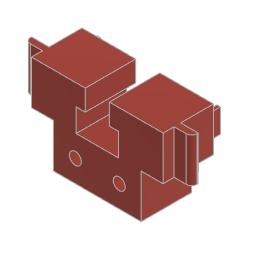
belt tensioner spacer (Autodesk Fusion 360 design; units mm, degrees)
Autodesk Fusion 360 part; units mm, degrees
sketch "Sketch1" plane through (0, 0, 0) normal (0, 1, 0) x (1, 0, 0)
  line L0 (0, 0) -> (0, -20) construction
  line L1 (0, -20) -> (30, -20)
  line L2 (30, -20) -> (30, 0)
  line L3 (30, 0) -> (20, 0)
  line L4 (20, 0) -> (20, 20)
  line L5 (20, 20) -> (0, 20)
  line L6 (-20, 0) -> (-20, 20)
  line L7 (-30, 0) -> (-20, 0)
  line L8 (-30, -20) -> (-30, 0)
  line L9 (-20, 20) -> (0, 20)
  line L10 (0, -20) -> (-30, -20)
  dimension "d1" = 20
  dimension "d2" = 30
  constraint coincident L0.start origin
  constraint vertical L0
  constraint perpendicular L0 L1
  constraint perpendicular L1 L2
  constraint perpendicular L2 L3
  constraint perpendicular L3 L4
  constraint perpendicular L4 L5
  constraint symmetric L1.start L0 L10.start
  constraint symmetric L0 L1.end L8.start
  constraint symmetric L0 L2.end L7.start
  constraint symmetric L0 L3.end L6.start
  constraint symmetric L0 L4.end L6.end
  constraint symmetric L0 L5.end L9.end
  measures "d1" distance of L0.start L0.end
  measures "d2" distance of L0.end L1.end
extrude "Extrude1" add sketch "Sketch1" along normal blind 15
sketch "Sketch2" plane through (0, 0, 0) normal (0, -1, 0) x (1, 0, 0)
  line L0 (30, 0) -> (30, 20)
  line L1 (30, 20) -> (-30, 20)
  line L2 (-30, 20) -> (-30, 0)
  line L3 (-30, 0) -> (-20, 0)
  line L4 (-20, 0) -> (-20, -20)
  line L5 (-20, -20) -> (20, -20)
  line L6 (20, -20) -> (20, 0)
  line L7 (20, 0) -> (30, 0)
  line L8 (30, 20) -> (38, 20)
  line L9 (38, 20) -> (38, 0)
  line L10 (38, 0) -> (30, 0)
  line L11 (30, 0) -> (30, 20)
  line L12 (-30, 20) -> (-38, 20)
  line L13 (-38, 20) -> (-38, 0)
  line L14 (-38, 0) -> (-30, 0)
  line L15 (-30, 0) -> (-30, 20)
  dimension "d5" = 8
  dimension "d6" = 8
  dimension "d7" = 20
  constraint horizontal L8
  constraint vertical L9
  constraint horizontal L10
  constraint vertical L11
  constraint coincident L0.end L1.start
  constraint horizontal L12
  constraint vertical L13
  constraint horizontal L14
  constraint vertical L15
  constraint coincident L1.end L2.start
  measures "d5" distance of L0.end L8.end
  measures "d6" distance of L1.end L12.end
  measures "d7" distance of L1.end L2.end
extrude "Extrude2" add sketch "Sketch2" along normal blind 3
sketch "Sketch3" plane through (0, -3, 0) normal (0, -1, 0) x (1, 0, 0)
  line L0 (38, 20) -> (-38, 20)
  line L1 (-38, 20) -> (-38, 0)
  line L2 (-38, 0) -> (-20, 0)
  line L3 (-20, 0) -> (-20, -20)
  line L4 (-20, -20) -> (20, -20)
  line L5 (20, -20) -> (20, 0)
  line L6 (20, 0) -> (38, 0)
  line L7 (38, 0) -> (38, 20)
  line L8 (-30, 20) -> (-30, 0)
  line L9 (0, 20) -> (-30, 20)
  line L10 (30, 20) -> (30, 0)
  line L11 (0, 20) -> (30, 20)
  line L12 (30, 0) -> (20, 0)
  line L13 (20, 0) -> (20, -20)
  line L14 (20, -20) -> (0, -20)
  line L15 (-20, -20) -> (0, -20)
  line L16 (-20, 0) -> (-20, -20)
  line L17 (-30, 0) -> (-20, 0)
extrude "Extrude3" add sketch "Sketch3" along normal blind 5 contours L0 L2 L3 L4 L5 L6 L8 L9 L10 L11 L12 L13 L14 L15 L16 L17
fillet "Fillet1" radius 2.5 2 edges at (38, -3, 10) (-38, -3, 10)
sketch "Sketch4" plane through (0, -8, 0) normal (0, -1, 0) x (1, 0, 0)
  line L0 (30, 20) -> (-30, 20)
  line L1 (-30, 20) -> (-30, 0)
  line L2 (-30, 0) -> (-20, 0)
  line L3 (-20, 0) -> (-20, -20)
  line L4 (-20, -20) -> (20, -20)
  line L5 (20, -20) -> (20, 0)
  line L6 (20, 0) -> (30, 0)
  line L7 (30, 0) -> (30, 20)
  line L8 (-20, -10) -> (20, -10) construction
  line L9 (20, 0) -> (20, -20)
  line L10 (-5.5, 20) -> (0, 20)
  line L11 (0, 20) -> (0, 13.9)
  line L12 (0, 13.9) -> (-5.5, 13.9)
  line L13 (-5.5, 13.9) -> (-5.5, 20)
  line L14 (0, 13.9) -> (5.5, 13.9)
  line L15 (5.5, 13.9) -> (5.5, 20)
  line L16 (5.5, 20) -> (0, 20)
  line L17 (14.8575, 20) -> (-15.1425, 20)
  line L18 (-15.1425, 20) -> (-15.1425, 10.5)
  line L19 (-15.1425, 10.5) -> (14.8575, 10.5)
  line L20 (14.8575, 10.5) -> (14.8575, 20)
  line L21 (14.8575, 20) -> (-15.1425, 10.5) construction
  line L22 (-15.1425, 20) -> (14.8575, 10.5) construction
  line L23 (9.65, 0) -> (-9.65, 0)
  line L24 (-9.65, 0) -> (-9.65, 10.5)
  line L25 (-9.65, 10.5) -> (9.65, 10.5)
  line L26 (9.65, 10.5) -> (9.65, 0)
  line L27 (9.65, 0) -> (-9.65, 10.5) construction
  line L28 (-9.65, 0) -> (9.65, 10.5) construction
  line L29 (5.5, 13.9) -> (14.8575, 13.9)
  line L30 (-15.1425, 13.9) -> (-5.5, 13.9)
  line L31 (-5.5, 13.9) -> (-5.5, 10.5)
  line L32 (5.5, 13.9) -> (5.5, 10.5)
  point P0 (-10, -10)
  point P1 (10, -10)
  point P2 (-0.1425, 15.25)
  point P3 (0, 5.25)
  dimension "d14" = 10
  dimension "d15" = 10
  dimension "d19" = 5.5
  dimension "d20" = 6.1
  dimension "d21" = 24.5
  dimension "d37" = 30
  dimension "d38" = 9.5
  dimension "d39" = 19.3
  dimension "d40" = 10.5
  constraint midpoint L3 L8.start
  constraint midpoint L5 L8.end
  constraint coincident L8 P0
  constraint coincident L8 P1
  constraint horizontal L10
  constraint vertical L11
  constraint horizontal L12
  constraint vertical L13
  constraint coincident L0 L10.start
  constraint symmetric L10.start L11 L15.end
  constraint symmetric L10.end L11 L16.end
  constraint symmetric L12.start L11 L14.start
  constraint symmetric L12.end L11 L14.end
  constraint horizontal L17
  constraint perpendicular L17 L18
  constraint parallel L17 L19
  constraint parallel L18 L20
  constraint coincident L21 P2
  constraint coincident L22 P2
  constraint collinear L0 L17
  constraint horizontal L23
  constraint perpendicular L23 L24
  constraint parallel L23 L25
  constraint parallel L24 L26
  constraint coincident L27 P3
  constraint coincident L28 P3
  constraint collinear L19 L25
  constraint coincident L20 L29.end
  constraint perpendicular L20 L29
  constraint coincident L18 L30.start
  constraint perpendicular L13 L30
  constraint coincident L25 L31.end
  constraint coincident L19 L32.end
  constraint vertical L32
  constraint vertical L31
  measures "d14" distance of L8.start P0
  measures "d15" distance of P1 L9
  measures "d19" distance of L11.end L12.end
  measures "d20" distance of L10.start L12.end
  measures "d21" distance of L0.end L13
  measures "d37" distance of L18.end L19.end
  measures "d38" distance of L17.end L18.end
  measures "d39" distance of L24.end L25.end
  measures "d40" distance of L23.end L24.end
hole "Hole1" at (10, -8, -10) at (-10, -8, -10) direction (0, 1, 0) diameter 5.5 end through all
extrude "Extrude4" cut sketch "Sketch4" against normal through all contours L0 L11 L14 L15 L16 L17 | L0 L10 L11 L12 L13 L17 | L12 L14 L19 L25 L31 L32 | L19 L23 L24 L25 L26
sketch "Sketch5" plane through (0, 15, 0) normal (0, 1, 0) x (-1, 0, 0)
  line L0 (-5.5, 20) -> (-30, 20)
  line L1 (-30, 20) -> (-30, 0)
  line L2 (-30, 0) -> (-20, 0)
  line L3 (-20, 0) -> (-20, -20)
  line L4 (-20, -20) -> (20, -20)
  line L5 (20, -20) -> (20, 0)
  line L6 (20, 0) -> (30, 0)
  line L7 (30, 0) -> (30, 20)
  line L8 (30, 20) -> (5.5, 20)
  circle A0 centre (-10, -10) radius 2.75
  circle A1 centre (10, -10) radius 2.75
  line L9 (0, 13.9) -> (0, -20) construction
  line L10 (-20, -10) -> (20, -10) construction
  line L11 (-16.55, -15.425) -> (-18.15, -15.425)
  line L12 (-18.15, -15.425) -> (-18.15, -4.575)
  line L13 (-18.15, -4.575) -> (-16.55, -4.575)
  line L14 (-16.55, -4.575) -> (-16.55, -15.425)
  line L15 (-16.55, -15.425) -> (-18.15, -4.575) construction
  line L16 (-18.15, -15.425) -> (-16.55, -4.575) construction
  line L17 (-13.95, -12.825) -> (-16.55, -12.825)
  line L18 (-16.55, -12.825) -> (-16.55, -7.175)
  line L19 (-16.55, -7.175) -> (-13.95, -7.175)
  line L20 (-13.95, -7.175) -> (-13.95, -12.825)
  line L21 (-13.95, -12.825) -> (-16.55, -7.175) construction
  line L22 (-16.55, -12.825) -> (-13.95, -7.175) construction
  line L23 (-16.55, -4.575) -> (-13.95, -7.175)
  line L24 (-13.95, -12.825) -> (-16.55, -15.425)
  line L25 (18.15, -4.575) -> (16.55, -4.575)
  line L26 (16.55, -4.575) -> (13.95, -7.175)
  line L27 (13.95, -7.175) -> (13.95, -12.825)
  line L28 (13.95, -12.825) -> (16.55, -15.425)
  line L29 (16.55, -15.425) -> (18.15, -15.425)
  line L30 (18.15, -15.425) -> (18.15, -4.575)
  line L31 (-30, 10) -> (30, 10) construction
  line L32 (-26.55, 4.575) -> (-28.15, 4.575)
  line L33 (-28.15, 4.575) -> (-28.15, 15.425)
  line L34 (-28.15, 15.425) -> (-26.55, 15.425)
  line L35 (-26.55, 15.425) -> (-26.55, 4.575)
  line L36 (-26.55, 4.575) -> (-28.15, 15.425) construction
  line L37 (-28.15, 4.575) -> (-26.55, 15.425) construction
  line L38 (-23.95, 7.175) -> (-26.55, 7.175)
  line L39 (-26.55, 7.175) -> (-26.55, 12.825)
  line L40 (-26.55, 12.825) -> (-23.95, 12.825)
  line L41 (-23.95, 12.825) -> (-23.95, 7.175)
  line L42 (-23.95, 7.175) -> (-26.55, 12.825) construction
  line L43 (-26.55, 7.175) -> (-23.95, 12.825) construction
  line L44 (-23.95, 12.825) -> (-26.55, 15.425)
  line L45 (-23.95, 7.175) -> (-26.55, 4.575)
  line L46 (23.95, 7.175) -> (26.55, 4.575)
  line L47 (23.95, 12.825) -> (23.95, 7.175)
  line L48 (23.95, 12.825) -> (26.55, 15.425)
  line L49 (28.15, 15.425) -> (26.55, 15.425)
  line L50 (28.15, 4.575) -> (28.15, 15.425)
  line L51 (26.55, 4.575) -> (28.15, 4.575)
  line L52 (5.5, 10.5) -> (9.65, 10.5)
  line L53 (9.65, 10.5) -> (9.65, 0)
  line L54 (9.65, 0) -> (-9.65, 0)
  line L55 (-9.65, 0) -> (-9.65, 10.5)
  line L56 (-9.65, 10.5) -> (-5.5, 10.5)
  line L57 (-5.5, 10.5) -> (-5.5, 20)
  line L58 (5.5, 20) -> (5.5, 10.5)
  point P0 (-17.35, -10)
  point P1 (-15.25, -10)
  point P2 (-27.35, 10)
  point P3 (-25.25, 10)
  dimension "d24" = 1.6
  dimension "d25" = 10.85
  dimension "d26" = 1.85
  dimension "d28" = 5.65
  dimension "d31" = 45
  dimension "d32" = 1.6
  dimension "d33" = 10.85
  dimension "d34" = 5.65
  dimension "d35" = 45
  dimension "d36" = 1.85
  constraint midpoint L4 L9.end
  constraint midpoint L3 L10.start
  constraint midpoint L5 L10.end
  constraint horizontal L11
  constraint perpendicular L11 L12
  constraint parallel L11 L13
  constraint parallel L12 L14
  constraint coincident L15 P0
  constraint coincident L16 P0
  constraint coincident L10 P0
  constraint horizontal L17
  constraint perpendicular L17 L18
  constraint parallel L17 L19
  constraint parallel L18 L20
  constraint coincident L21 P1
  constraint coincident L22 P1
  constraint coincident L10 P1
  constraint collinear L14 L18
  constraint symmetric L9 L11.start L28.end
  constraint symmetric L9 L11.end L29.end
  constraint symmetric L9 L12.end L25.start
  constraint symmetric L9 L13.end L25.end
  constraint symmetric L9 L17.start L27.end
  constraint symmetric L9 L19.end L26.end
  constraint midpoint L1 L31.start
  constraint midpoint L7 L31.end
  constraint horizontal L32
  constraint perpendicular L32 L33
  constraint parallel L32 L34
  constraint parallel L33 L35
  constraint coincident L36 P2
  constraint coincident L37 P2
  constraint coincident L31 P2
  constraint horizontal L38
  constraint perpendicular L38 L39
  constraint parallel L38 L40
  constraint parallel L39 L41
  constraint coincident L42 P3
  constraint coincident L43 P3
  constraint coincident L31 P3
  constraint collinear L35 L39
  constraint symmetric L9 L32.start L46.end
  constraint symmetric L9 L32.end L50.start
  constraint symmetric L9 L33.end L49.start
  constraint symmetric L9 L34.end L48.end
  constraint symmetric L9 L38.start L46.start
  constraint symmetric L9 L40.end L47.start
  measures "d24" distance of L12.end L13.end
  measures "d25" distance of L11.end L12.end
  measures "d26" distance of L3 L12
  measures "d28" distance of L17.end L18.end
  measures "d31" angle of L14 L23
  measures "d32" distance of L33.end L34.end
  measures "d33" distance of L32.end L33.end
  measures "d34" distance of L38.end L39.end
  measures "d35" angle of L35 L44
  measures "d36" distance of L1 L33
extrude "Extrude5" add sketch "Sketch5" along normal blind 5 contours L11 L12 L13 L14 L18 | L14 L17 L24 | L14 L17 L18 L19 L20 | L14 L19 L23 | L25 L26 L27 L28 L29 L30 | L32 L33 L34 L35 L39 | L35 L38 L45 | L35 L38 L39 L40 L41 | L35 L40 L44 | L46 L47 L48 L49 L50 L51
